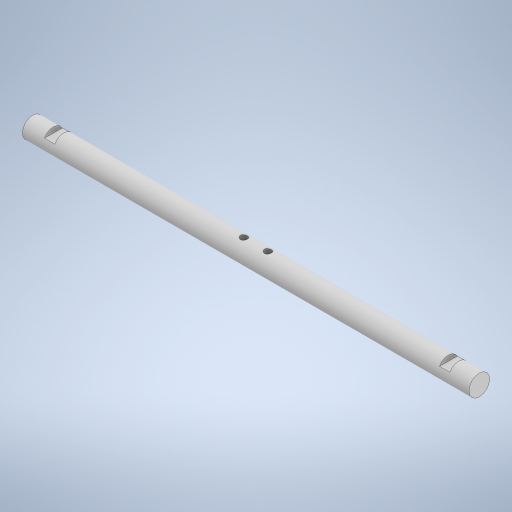
# Autodesk Inventor part: base_axis_12mm
Saved by Autodesk Inventor 2024 (Build 280153000, 153)
## iProperties
Created: 2025-12-09
Part Number: base_axis_12mm
Material: Generic
Document SubType Name: Modeling
Designer: schar
Density: 1 g/cm^3
Appearance: Default
Author: schar
Autodesk Inventor part; units mm, degrees
ref_plane "YZ Plane" through (0, 0, 0) normal (1, 0, 0) x (0, 1, 0)
ref_plane "XZ Plane" through (0, 0, 0) normal (0, 1, 0) x (-1, 0, 0)
ref_plane "XY Plane" through (0, 0, 0) normal (0, 0, 1) x (1, 0, 0)
sketch "Sketch1" plane through (0, 0, 0) normal (1, 0, 0) x (0, 1, 0)
  circle A0 centre (0, 0) radius 6
  dimension "d0" = 12
  constraints: 1 centre point, 1 coincident
  measures "d0" diameter of A0
extrude "Extrusion1" add sketch "Sketch1" along normal mid plane 260
sketch "Sketch2" plane through (0, 0, 0) normal (0, 0, 1) x (1, 0, 0)
  line L0 (-130, 6) -> (-130, -6) projected
  line L1 (-130, 0) -> (-115, 0)
  line L2 (-115, 0) -> (-115, 6)
  line L3 (130, -6) -> (130, 6) projected
  line L4 (130, 0) -> (115, 0)
  line L5 (115, 0) -> (115, 6)
  line L6 (112, 9) -> (118, 9)
  line L7 (118, 9) -> (118, 3)
  line L8 (118, 3) -> (112, 3)
  line L9 (112, 3) -> (112, 9)
  line L10 (112, 9) -> (118, 3) construction
  line L11 (118, 9) -> (112, 3) construction
  line L12 (-118, 9) -> (-112, 9)
  line L13 (-112, 9) -> (-112, 3)
  line L14 (-112, 3) -> (-118, 3)
  line L15 (-118, 3) -> (-118, 9)
  line L16 (-118, 9) -> (-112, 3) construction
  line L17 (-112, 9) -> (-118, 3) construction
  point P0 (0, 0)
  dimension "d3" = 15
  dimension "d4" = 15
  dimension "d5" = 6
  dimension "d6" = 6
  constraints: 32 end point, 6 midpoint, 4 horizontal, 4 parallel, 3 perpendicular, 1 vertical
  measures "d3" distance of L1.start L1.end
  measures "d4" distance of L4.start L4.end
  measures "d5" distance of L7.end L8.end
  measures "d6" distance of L13.end L14.end
extrude "Extrusion2" cut sketch "Sketch2" along normal mid plane 20
sketch "Sketch3" plane through (0, 0, 0) normal (0, 1, 0) x (-1, 0, 0)
  line L0 (-130, 6) -> (-130, -6) projected
  line L1 (-130, -6) -> (-5, -6)
  line L2 (130, -6) -> (-130, -6) projected
  line L3 (-5, -6) -> (-5, 0)
  line L4 (130, 6) -> (-130, 6) projected
  line L5 (-5, 0) -> (5, 0)
  line L6 (5, 0) -> (7, 0)
  line L7 (-5, 0) -> (-7, 0)
  circle A0 centre (7, 0) radius 2
  circle A1 centre (-7, 0) radius 2
  point P0 (0, 0)
  dimension "d9" = 125
  dimension "d10" = 10
  dimension "d11" = 2
  dimension "d12" = 2
  constraints: 10 end point, 2 coincident, 2 horizontal, 2 horizontal alignment, 2 perpendicular, 1 point on line, 4 other
  measures "d9" distance of L0.end L1.end
  measures "d10" distance of L3.end L5.end
  measures "d11" distance of L5.end L6.end
  measures "d12" distance of L3.end L7.end
extrude "Extrusion3" cut sketch "Sketch3" along normal blind 10
thread "Thread1" size "M4x0.7" class "6H" standard "ANSI Metric M Profile" full length
thread "Thread2" size "M4x0.7" class "6H" standard "ANSI Metric M Profile" full length
body "Solid1"
